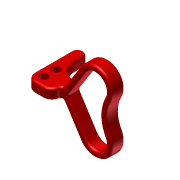
# Autodesk Inventor part: parte_4
Saved by Autodesk Inventor 2012 SP2 (Build 160219200, 219)
## iProperties
Created: 2015-05-26
Part Number: parte_4
Material: Aço carbono
Document SubType Name: Modeling
Designer: Projeto02
Density: 7.87 g/cm^3
Mass: 418.933 g
Surface Area: 172.237 cm^2
Volume: 53.2317 cm^3
Author: Projeto02
Autodesk Inventor part; units mm, degrees
ref_plane "YZ Plane" through (0, 0, 0) normal (1, 0, 0) x (0, 1, 0)
ref_plane "XZ Plane" through (0, 0, 0) normal (0, 1, 0) x (-1, 0, 0)
ref_plane "XY Plane" through (0, 0, 0) normal (0, 0, 1) x (1, 0, 0)
sketch "Esboço1" plane through (0, 0, 0) normal (0, 0, 1) x (1, 0, 0)
  circle A0 centre (0, 0) radius 5.5
  circle A1 centre (0, 16.5) radius 5.5
  line L0 (-12, 0) -> (-12, 56.5)
  line L1 (0, 16.5) -> (-12, 16.5)
  line L2 (3, 56.5) -> (3, 38.3192)
  line L3 (-12, 56.5) -> (3, 56.5)
  arc A2 (3, 38.3192) -> (23, 17.5) centre (23.836, 38.3192) ccw
  line L4 (0, -12) -> (11, -12)
  arc A3 (-12, 0) -> (0, -12) centre (0, 0) ccw
  arc A4 (11, -12) -> (23, 0) centre (11, 0) ccw
  line L5 (23, 17.5) -> (25, 17.5)
  line L6 (25, 17.5) -> (25, 0)
  line L7 (25, 0) -> (23, 0)
  dimension "d0" = 11
  dimension "d1" = 11
  dimension "d2" = 16.5
  dimension "d3" = 12
  dimension "d4" = 12
  dimension "d5" = 40
  dimension "d6" = 15
  dimension "d9" = 12
  dimension "d27" = 20.836
  dimension "d30" = 17.5
  dimension "d31" = 2
  constraints: 16 end point, 6 point on circle, 5 centre point, 5 perpendicular, 3 tangent, 2 coincident, 2 vertical alignment, 1 parallel, 1 point on line
  measures "d0" diameter of A0
  measures "d1" diameter of A1
  measures "d2" distance of L1.start A0.centre
  measures "d3" distance from line of L1.start L0
  measures "d4" distance from line of point (0, 0) L0
  measures "d5" distance from line of L0.end L1
  measures "d6" distance between parallel lines of L2 L0
  measures "d9" radius of A4
  measures "d27" distance from line of A2.centre L2
  measures "d30" distance of L7.end L5.start
  measures "d31" distance of L5.start L5.end
extrude "Extrusão1" add sketch "Esboço1" along normal mid plane 14
fillet "Arredondamento1" radius 7 2 edges at (-12, 56.5, 0) (3, 56.5, 0)
sketch "Esboço3" plane through (0, 0, 0) normal (0, 1, 0) x (-1, 0, 0)
  arc A0 (-54.8491, 38.0595) -> (-80.6684, 22.8172) centre (-67.5, 30) ccw
  arc A1 (-80.6684, -22.8172) -> (-54.8491, -38.0595) centre (-67.5, -30) ccw
  arc A2 (-87.6367, -19.0163) -> (-48.1547, -42.3243) centre (-67.5, -30) ccw
  arc A3 (-87.6367, -19.0163) -> (-87.6367, 19.0163) centre (-122.5, 0) ccw
  arc A4 (-80.6684, -22.8172) -> (-80.6684, 22.8172) centre (-122.5, 0) ccw
  line L0 (-54.8491, -38.0595) -> (-30.6026, 0)
  line L1 (-54.8491, 38.0595) -> (-30.6026, 0)
  arc A5 (-48.1547, 42.3243) -> (-87.6367, 19.0163) centre (-67.5, 30) ccw
  line L2 (-25.6506, -7) -> (-25, -7)
  line L3 (-25.6506, 7) -> (-25, 7)
  line L4 (-25, 7) -> (-25, -7)
  line L5 (-25, 7) -> (-25, -7) projected
  line L6 (-23, -7) -> (-25, -7) projected
  line L7 (-25, 7) -> (-23, 7) projected
  line L8 (-25.6506, 7) -> (-48.1547, 42.3243)
  line L9 (-25.6506, -7) -> (-48.1547, -42.3243)
  point P0 (0, 0)
  dimension "d13" = 30
  dimension "d14" = 30
  dimension "d15" = 60
  dimension "d16" = 30
  dimension "d17" = 67.5
  dimension "d19" = 7.9375
  dimension "d20" = 55
  constraints: 14 end point, 12 point on circle, 6 centre point, 6 tangent, 3 coincident, 3 collinear, 2 horizontal alignment, 2 parallel, 1 vertical alignment
  measures "d13" diameter of A1
  measures "d14" diameter of A0
  measures "d15" distance of A0.centre A1.centre
  measures "d16" vertical distance of point (0, 0) A0.centre
  measures "d17" horizontal distance of point (0, 0) A0.centre
  measures "d19" radial gap between concentric circles of A2 A1
  measures "d20" horizontal distance of A0.centre A4.centre
extrude "Extrusão3" add sketch "Esboço3" along normal blind 17.5
fillet "Arredondamento4" radius 2.943 1 edges at (23, 0, 0)
fillet "Arredondamento5" radius 4 3 edges at (30.6026, 8.75, 0) (25.6506, 8.75, -7) (25.6506, 8.75, 7)
fillet "Arredondamento6" radius 3 50 edges at (26.3035, 0, -8.1906) (24.4665, -0.2486, -7.1297) (23.0183, -1.6263, -7) (18.6039, -9.2833, -7) (5.5, -12, -7) (-8.4853, -8.4853, -7) (-12, 24.75, -7) (-9.9497, 54.4497, -7) (-4.5, 56.5, -7) (0.9497, 54.4497, -7) (3, 43.9096, -7) (8.8101, 23.8845, -7) (79.1607, 0, -49.7524) (82.7877, 0, 0) (79.1607, 0, 49.7524) (37.4922, 0, 25.5876) (26.3035, 0, 8.1906) (24.4665, -0.2486, 7.1297) (23.0183, -1.6263, 7) (18.6039, -9.2833, 7) (5.5, -12, 7) (-8.4853, -8.4853, 7) (-12, 24.75, 7) (-9.9497, 54.4497, 7) (-4.5, 56.5, 7) (0.9497, 54.4497, 7) (3, 43.9096, 7) (8.8101, 23.8845, 7) (37.4922, 0, -25.5876) (79.1607, 17.5, -49.7524) (82.7877, 17.5, 0) (79.1607, 17.5, 49.7524) (37.4922, 17.5, 25.5876) (25.3801, 17.5, 7.4931) (23.2281, 17.5, 7) (25.3801, 17.5, -7.4931) (23.2281, 17.5, -7) (37.4922, 17.5, -25.5876) (31.3453, 0, 0) (43.4104, 0, 20.1043) (75.1255, 0, 42.9171) (74.8502, 0, 0) (75.1255, 0, -42.9171) (43.4104, 0, -20.1043) (31.3453, 17.5, 0) (43.4104, 17.5, -20.1043) (75.1255, 17.5, -42.9171) (74.8502, 17.5, 0) (75.1255, 17.5, 42.9171) (43.4104, 17.5, 20.1043)
equation "\"d4\" = d3"
equation "\"d14\" = d13"
equation "\"d16\" = d14"
equation "\"d19\" = d18"
equation "\"d18\" = 7.9375"
